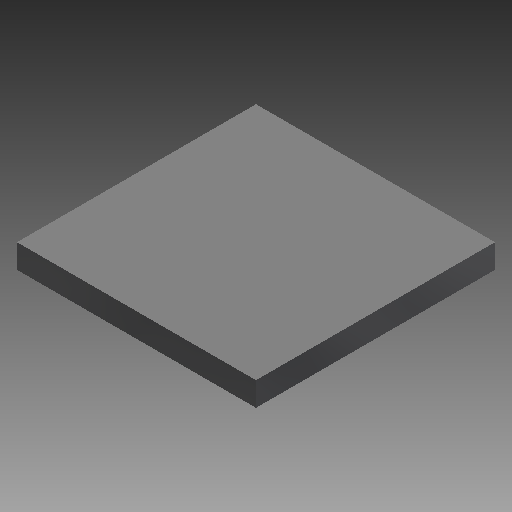
# Autodesk Inventor part: Thermal pad .100
Saved by Autodesk Inventor 2017 (Build 210142000, 142)
## iProperties
Created: 2016-03-02
Part Number: Thermal pad .100
Material: Rubber, Silicone
Document SubType Name: Modeling
Designer: rtreacy
Density: 1 g/cm^3
Appearance: Rubber - Black - Version 1.1
Description: .125 thickness important
Vendor: Bergquist
Stock Number: HC 3.0-0.125-02-0404
Author: rtreacy
Autodesk Inventor part; units mm, degrees
ref_plane "YZ Plane" through (0, 0, 0) normal (1, 0, 0) x (0, 1, 0)
ref_plane "XZ Plane" through (0, 0, 0) normal (0, 1, 0) x (-1, 0, 0)
ref_plane "XY Plane" through (0, 0, 0) normal (0, 0, 1) x (1, 0, 0)
sketch "Sketch1" plane through (0, 0, 0) normal (0, 1, 0) x (-1, 0, 0)
  line L0 (-26.5616, 27.4134) -> (-1.1616, 27.4134)
  line L1 (-1.1616, 27.4134) -> (-1.1616, 2.0134)
  line L2 (-1.1616, 2.0134) -> (-26.5616, 2.0134)
  line L3 (-26.5616, 2.0134) -> (-26.5616, 27.4134)
  point P0 (0, 0)
  dimension "d0" = 25.4
  dimension "d2" = 25.4
  constraints: 8 end point, 2 parallel, 1 horizontal, 1 perpendicular
  measures "d0" distance of L2.end L0.start
  measures "d2" distance of L0.end L0.start
extrude "Extrusion1" add sketch "Sketch1" along normal blind 2.54
body "Solid1"
